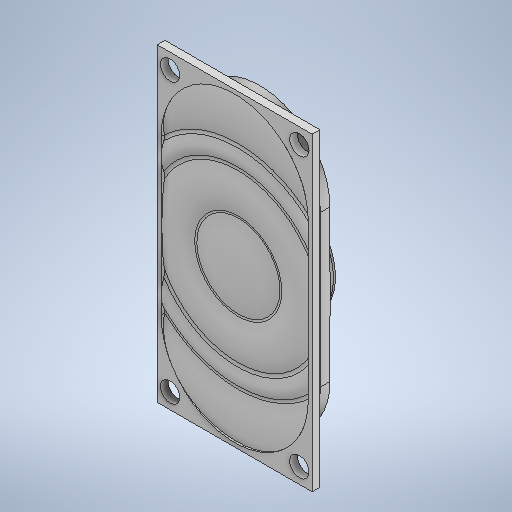
# Autodesk Inventor part: Speaker 2040 8Ohm 2W
Saved by Autodesk Inventor 2025 (Build 290162000, 162)
## iProperties
Created: 2025-09-27
Part Number: Speaker 2040 8Ohm 2W
Material: Generic
Document SubType Name: Modeling
Designer: naufal
Density: 1 g/cm^3
Appearance: Default
Author: naufal
Autodesk Inventor part; units mm, degrees
ref_plane "YZ Plane" through (0, 0, 0) normal (1, 0, 0) x (0, 1, 0)
ref_plane "XZ Plane" through (0, 0, 0) normal (0, 1, 0) x (-1, 0, 0)
sketch "Sketch1" plane through (0, 0, 0) normal (0, 0, 1) x (1, 0, 0)
  line L0 (17.0475, 24.231) -> (71.7228, 24.231) construction
  line L1 (71.7228, 24.231) -> (71.7228, -21.7333) construction
  line L2 (71.7228, -21.7333) -> (17.0475, -21.7333) construction
  line L3 (17.0475, -21.7333) -> (17.0475, 24.231) construction
  line L4 (10, -20) -> (-10, -20)
  line L5 (-10, -20) -> (-10, 20)
  line L6 (-10, 20) -> (10, 20)
  line L7 (10, 20) -> (10, -20)
  line L8 (10, -20) -> (-10, 20) construction
  line L9 (-10, -20) -> (10, 20) construction
  line L10 (-9.5, -10) -> (-9.5, 10)
  line L11 (9.5, 10) -> (9.5, -10)
  line L12 (9.5, -10) -> (-9.5, 10) construction
  line L13 (-9.5, -10) -> (9.5, 10) construction
  line L14 (-7, -6.5) -> (-7, 6.5)
  line L15 (7, 6.5) -> (7, -6.5)
  line L16 (7, -6.5) -> (-7, 6.5) construction
  line L17 (-7, -6.5) -> (7, 6.5) construction
  line L18 (-6, -5) -> (-6, 5)
  line L19 (6, 5) -> (6, -5)
  line L20 (6, -5) -> (-6, 5) construction
  line L21 (-6, -5) -> (6, 5) construction
  arc A0 (9.5, 10) -> (-9.5, 10) centre (0, 10) ccw
  arc A1 (7, 6.5) -> (-7, 6.5) centre (0, 6.5) ccw
  arc A2 (6, 5) -> (-6, 5) centre (0, 5) ccw
  arc A3 (-9.5, -10) -> (9.5, -10) centre (0, -10) ccw
  arc A4 (-6, -5) -> (6, -5) centre (0, -5) ccw
  arc A5 (-7, -6.5) -> (7, -6.5) centre (0, -6.5) ccw
  circle A6 centre (8.35, 18) radius 1.25
  circle A7 centre (-8.35, 18) radius 1.25
  circle A8 centre (8.35, -18) radius 1.25
  circle A9 centre (-8.35, -18) radius 1.25
  circle A10 centre (0, 0) radius 5.5
  constraints: 36 end point, 12 point on circle, 11 centre point, 5 parallel, 1 horizontal, 1 midpoint, 1 perpendicular, 2 other
extrude "Extrusion1" add sketch "Sketch1" against normal blind 1 contours L4 L5 L6 L7
extrude "Extrusion2" add sketch "Sketch1" against normal blind 1 separate body contours L10 A0 L11 A3 | L14 A1 L15 A5 | L18 A2 L19 A4 | A10
ref_plane "Work Plane5" through (0, -20, 0) normal (-1, 0, 0) x (0, 0, 1)
sketch "Sketch4" plane through (0, -20, 0) normal (-1, 0, 0) x (0, 0, 1)
  line L0 (0, 14.5) -> (0, 25.5) projected
  line L1 (0, 9) -> (0, 15) projected
  line L2 (0, 6.5) -> (0, 13.5) projected
  line L3 (0, 0.5) -> (0, 10) projected
  line L4 (0, 33.5) -> (-0.5, 33.5)
  line L5 (-1, 40) -> (-1, 0) projected
  line L6 (0, 31) -> (-0.5, 31)
  line L7 (0, 25.5) -> (-0.5, 25.5)
  line L8 (0, 14.5) -> (-0.5, 14.5)
  line L9 (0, 9) -> (-0.5, 9)
  line L10 (0, 6.5) -> (-0.5, 6.5)
  line L11 (0, 39.5) -> (-0.25, 39.5)
  line L12 (-1, 39.5) -> (0, 39.5) projected
  line L13 (0, 0.5) -> (-0.25, 0.5)
  line L14 (-1, 0.5) -> (0, 0.5) projected
  arc A0 (-0.4307, 33.7476) -> (-0.25, 39.5) centre (-12.5515, 37.0074) ccw
  arc A1 (-0.3403, 31.1928) -> (-0.351, 33.322) centre (-1.8125, 32.25) ccw
  arc A2 (-0.4547, 25.6236) -> (-0.408, 30.7417) centre (-7.8125, 28.25) ccw
  arc A3 (-0.5, 14.5) -> (-0.476, 25.3675) centre (-30.5, 20) ccw
  line L15 (0, 39.5) -> (1, 39.5)
  line L16 (1, 39.5) -> (1, 20)
  line L17 (1, 20) -> (0, 20)
  arc A4 (-0.4307, 33.7476) -> (-0.351, 33.322) centre (0.0522, 33.6177) ccw
  arc A5 (-0.3403, 31.1928) -> (-0.408, 30.7417) centre (0.0659, 30.9012) ccw
  arc A6 (-0.4547, 25.6236) -> (-0.476, 25.3675) centre (0.0162, 25.4555) ccw
  point P0 (0, 30)
  point P1 (0, 26.5)
  point P2 (0, 25)
  point P3 (0, 15)
  point P4 (0, 13.5)
  point P5 (0, 10)
  dimension "d57" = 0.5
  dimension "d58" = 0.25
  dimension "d59" = 0.25
  dimension "d60" = 1
  dimension "d61" = 0.5
  constraints: 22 end point, 20 point on circle, 8 coincident, 7 centre point, 7 tangent, 6 horizontal, 2 equal radius, 2 perpendicular, 2 point on line
  measures "d57" distance of L4.start L4.end
  measures "d58" distance of L11.start L11.end
  measures "d59" distance of L13.start L13.end
  measures "d60" distance of L12.end L15.end
  measures "d61" radius of A4
revolve "Revolution1" cut sketch "Sketch4" angle 360 about axis through (0, 0, 1) along (0, 0, -1) bodies 2 contours A3 A6 L7 L0 | L0 L7 A6 A2 A5 A1 A4 A0 L11 L15 L16 L17
combine bodies "Combine1" operation type add bodies to combine 1 2
sketch "Sketch5" plane through (10, 20, -1) normal (0, 0, -1) x (-1, 0, 0)
  line L0 (20, -40) -> (0, -40)
  line L1 (0, -40) -> (0, 0)
  line L2 (0, 0) -> (20, 0)
  line L3 (20, 0) -> (20, -40)
  line L4 (20, -40) -> (0, 0) construction
  line L5 (0, -40) -> (20, 0) construction
  line L6 (19.5, -30) -> (0.5, -10) construction
  line L7 (0.5, -30) -> (19.5, -10) construction
  line L8 (17, -26.5) -> (3, -13.5) construction
  line L9 (3, -26.5) -> (17, -13.5) construction
  line L10 (16, -25) -> (4, -15) construction
  line L11 (4, -25) -> (16, -15) construction
  circle A0 centre (18.35, -2) radius 1.25
  circle A1 centre (1.65, -2) radius 1.25
  circle A2 centre (1.65, -38) radius 1.25
  circle A3 centre (18.35, -38) radius 1.25
  circle A4 centre (1.65, -2) radius 1.25 projected
  circle A5 centre (10, -20) radius 7.5
  line L12 (10, -1.1873) -> (10, -38.8127) construction
  line L13 (19.046, -10.2333) -> (19.046, -29.7667)
  line L14 (0.954, -29.7667) -> (0.954, -10.2333)
  arc A6 (19.046, -10.2333) -> (0.954, -10.2333) centre (10, -10.2333) ccw
  arc A7 (0.954, -29.7667) -> (19.046, -29.7667) centre (10, -29.7667) ccw
  arc A8 (6.1956, -32.5525) -> (13.9735, -32.7216) centre (10.2353, -25.703) ccw
  line L15 (6.1956, -32.5525) -> (3.8066, -36.36)
  line L16 (13.9735, -32.7216) -> (16.5196, -36.0376)
  point P0 (10, -20)
  point P1 (10, -20)
  point P2 (10, -20)
  dimension "d64" = 15
  constraints: 36 end point, 10 point on circle, 8 centre point, 4 tangent, 3 parallel, 2 point on line, 1 horizontal, 1 midpoint, 1 perpendicular, 1 vertical
  measures "d64" diameter of A5
extrude "Extrusion3" add sketch "Sketch5" along normal blind 1 contours A7 L15 A8 L16 bodies 1
extrude "Extrusion4" add sketch "Sketch5" along normal blind 2.25 contours L13 A7 L16 A8 L15 L14 A6 bodies 1
extrude "Extrusion5" add sketch "Sketch5" along normal blind 4.5 contours A5 bodies 1
fillet "Fillet1" radius 2 1 edges at (7.5, 0, -3.25)
fillet "Fillet2" radius 1 4 edges at (9.046, 0, -1) (0, 18.8127, -1) (-9.046, 0, -1) (0, -18.8127, -1)
body "Solid1"
